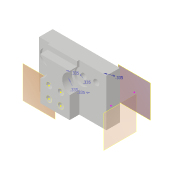
# Autodesk Inventor part: CollectorArmRollerSupportRight
Saved by Autodesk Inventor 2018 (Build 220112000, 112)
## iProperties
Created: 2018-12-16
Part Number: CollectorArmRollerSupportRight
Material: Generic
Document SubType Name: Modeling
Designer: ball
Density: 1 g/cm^3
Appearance: Default
Author: ball
Autodesk Inventor part; units mm, degrees
ref_plane "Work Plane5" through (0, 0, 0) normal (0, 0, 1) x (1, 0, 0)
sketch "Sketch1" plane through (0, 0, 0) normal (0, 0, 1) x (1, 0, 0)
  line L0 (-46.1271, -22.5825) -> (-26.1271, -22.5825) construction
  line L1 (-9.7566, 12.6962) -> (-9.7566, -12.6962) construction
  line L2 (-26.1271, 20.28) -> (-46.1271, 20.28) construction
  circle A0 centre (-49.897, 0) radius 1.778
  arc A1 (-26.7903, 1.7468) -> (-25.506, 1.3298) centre (-26.6476, 0) ccw construction
  circle A2 centre (-49.897, 0) radius 1.905
  circle A3 centre (-26.6476, 0) radius 1.905
  line L3 (-52.9366, 6.2882) -> (-52.9366, -15.9368)
  line L4 (-55.4766, 6.2882) -> (-55.4766, -15.9368) construction
  line L5 (-9.7566, -22.5825) -> (-55.4766, -22.5825)
  line L6 (-55.4766, -22.5825) -> (-55.4766, 20.28)
  line L7 (-55.4766, 20.28) -> (-9.7566, 20.28)
  line L8 (-9.7566, 20.28) -> (-9.7566, -22.5825)
  circle A4 centre (-16.5926, 2.1082) radius 2.15 construction
  circle A5 centre (-16.5926, 2.1082) radius 1.9939
  point P0 (0, 0)
  dimension "d0" = 3.81
  dimension "d1" = 3.81
  dimension "d2" = 2.54
  dimension "d3" = 3.9878
  constraints: 18 end point, 6 centre point, 3 coincident, 3 horizontal, 3 parallel, 2 point on circle, 2 vertical, 1 perpendicular, 16 other
  measures "d0" diameter of A2
  measures "d1" diameter of A3
  measures "d2" distance between parallel lines of L3 L4
  measures "d3" diameter of A5
ref_plane "Work Plane2" through (-20.9694, -2.2685, 9.225) normal (0, 0, -1) x (0.1078, 0.9942, 0)
extrude "Extrusion1" add sketch "Sketch1" along normal up to surface (9.225 mm away) contours A2 | L5 L6 L7 L8
ref_plane "Work Plane3" through (-49.3551, -24.0887, 15.745) normal (0, 0, -1) x (0, 1, 0)
ref_plane "Work Plane7" through (-55.4766, -22.5825, 9.225) normal (0, 0, 1) x (1, 0, 0)
sketch "Sketch3" plane through (-55.4766, -22.5825, 9.225) normal (0, 0, 1) x (1, 0, 0)
  line L0 (27.2386, 42.8625) -> (7.2386, 42.8625) projected
  arc A0 (27.2386, 28.0707) -> (27.2386, 14.6543) centre (29.2386, 21.3625) ccw projected
  line L1 (27.2386, 0) -> (27.2386, 14.6543) projected
  line L2 (7.2386, 14.6543) -> (7.2386, 0) projected
  line L3 (7.2386, 0) -> (27.2386, 0) projected
  arc A1 (7.2386, 14.6543) -> (7.2386, 28.0707) centre (5.2386, 21.3625) ccw projected
  line L4 (7.2386, 28.0707) -> (7.2386, 42.8625)
  line L5 (0, 42.8625) -> (45.72, 42.8625) projected
  line L6 (27.2386, 28.0707) -> (27.2386, 42.8625)
  point P0 (55.4766, 22.5825)
  constraints: 4 end point, 1 perpendicular, 1 vertical
ref_plane "Work Plane4" through (-51.466, -24.0887, 15.745) normal (0, 0, -1) x (0, 1, 0)
extrude "Extrusion3" add sketch "Sketch3" along normal up to surface (6.52 mm away)
ref_plane "Work Plane9" through (-55.4766, -22.5825, 9.225) normal (0, 0, 1) x (1, 0, 0)
sketch "Sketch4" plane through (-55.4766, -22.5825, 9.225) normal (0, 0, 1) x (1, 0, 0)
  circle A0 centre (5.5796, 22.5825) radius 1.778 projected
  circle A1 centre (5.5796, 22.5825) radius 1.905
  line L0 (7.2386, 28.0707) -> (7.2386, 42.8625) projected
  line L1 (7.2386, 42.8625) -> (0, 42.8625) projected
  line L2 (0, 42.8625) -> (0, 0) projected
  line L3 (0, 0) -> (7.2386, 0) projected
  line L4 (7.2386, 0) -> (7.2386, 14.6543) projected
  arc A2 (7.2386, 14.6543) -> (7.2386, 28.0707) centre (5.2386, 21.3625) ccw projected
  circle A3 centre (5.5796, 22.5825) radius 1.778 projected
  circle A4 centre (28.829, 22.5825) radius 1.9812 projected
  point P0 (55.4766, 22.5825)
  dimension "d18" = 3.81
  constraints: 1 centre point, 1 coincident
  measures "d18" diameter of A1
hole "Hole1" at (-49.897, 0, 9.225) at (-26.6476, 0, 9.225) direction (0, 0, -1) diameter 3.81 end through all counterbore diameter 10.16 counterbore depth 1.524
ref_plane "Work Plane8" through (-9.7566, -22.5825, 0) normal (1, 0, 0) x (0, 0, -1)
sketch "Sketch6" plane through (-9.7566, -22.5825, 0) normal (1, 0, 0) x (0, 0, -1)
  line L0 (-11.975, 30.2275) -> (-14.475, 30.2275) construction
  line L1 (-11.975, 39.7275) -> (-11.975, 30.2275) construction
  line L2 (31.025, 39.7275) -> (-11.975, 39.7275) construction
  line L3 (31.025, 38.4575) -> (-10.705, 38.4575) construction
  line L4 (-10.705, 32.1075) -> (-10.705, 28.9575) construction
  line L5 (-10.705, 28.9575) -> (-14.475, 28.9575) construction
  line L6 (-10.705, 28.9575) -> (-10.705, 32.1075)
  line L7 (0, 42.8625) -> (0, 0) projected
  line L8 (0, 32.1075) -> (0, 42.8625)
  line L9 (0, 42.8625) -> (-15.745, 42.8625)
  line L10 (-15.745, 42.8625) -> (-15.745, 28.9575)
  line L11 (-15.745, 28.9575) -> (-10.705, 28.9575)
  line L12 (3.1182, 32.1075) -> (5.3958, 32.1075) construction
  line L13 (-10.705, 32.1075) -> (0, 32.1075)
  point P0 (0, 22.5825)
  point P1 (0, 38.4575)
  dimension "d28" = 1.27
  constraints: 20 end point, 4 point on line, 3 collinear, 3 perpendicular, 1 horizontal, 2 other
  measures "d28" distance between parallel lines of L2 L3
extrude "Extrusion4" cut sketch "Sketch6" against normal through all
sketch "Sketch7" plane through (-48.238, -22.5825, 15.745) normal (0, 0, 1) x (1, 0, 0)
  circle A0 centre (6, 5.3625) radius 2 construction
  circle A1 centre (14, 5.3625) radius 2 construction
  arc A2 (7.4142, 14.7767) -> (4.5858, 11.9483) centre (6, 13.3625) ccw construction
  arc A3 (15.4142, 11.9483) -> (12.5858, 14.7767) centre (14, 13.3625) ccw construction
  point P0 (48.238, 22.5825)
sketch "Sketch9" plane through (0, 0, 0) normal (0, 0, -1) x (-1, 0, 0)
  arc A0 (43.6522, -10.6342) -> (40.8238, -7.8058) centre (42.238, -9.22) ccw construction
  arc A1 (35.6522, -7.8058) -> (32.8238, -10.6342) centre (34.238, -9.22) ccw construction
  circle A2 centre (42.238, -17.22) radius 2 construction
  circle A3 centre (34.238, -17.22) radius 2 construction
  point P0 (0, 0)
hole "Hole2" at (-34.238, -9.22, 0) at (-42.238, -9.22, 0) at (-42.238, -17.22, 0) at (-34.238, -17.22, 0) direction (0, 0, 1) diameter 3.9878 end through all
ref_plane "Work Plane6" through (0, 0, 0) normal (0, 0, -1) x (-1, 0, 0)
sketch "Sketch10" plane through (0, 0, 0) normal (0, 0, -1) x (-1, 0, 0)
  circle A0 centre (34.238, -9.22) radius 1.9939 construction
  circle A1 centre (42.238, -9.22) radius 1.9939 construction
  circle A2 centre (42.238, -17.22) radius 1.9939 construction
  circle A3 centre (34.238, -17.22) radius 1.9939 construction
  circle A4 centre (34.238, -9.22) radius 4.2545 construction
  circle A5 centre (42.238, -9.22) radius 4.2545 construction
  line L0 (34.238, -13.4745) -> (30.5535, -11.3472)
  line L1 (30.5535, -11.3472) -> (30.5535, -7.0927)
  line L2 (30.5535, -7.0927) -> (34.238, -4.9655)
  line L3 (34.238, -4.9655) -> (37.9225, -7.0927)
  line L4 (37.9225, -7.0927) -> (37.9225, -11.3472)
  line L5 (37.9225, -11.3472) -> (34.238, -13.4745)
  circle A6 centre (34.238, -17.22) radius 4.2545 construction
  circle A7 centre (42.238, -17.22) radius 4.2545 construction
  line L6 (38.4925, -17.22) -> (36.3652, -20.9045)
  line L7 (36.3652, -20.9045) -> (32.1107, -20.9045)
  line L8 (32.1107, -20.9045) -> (29.9835, -17.22)
  line L9 (29.9835, -17.22) -> (32.1107, -13.5355)
  line L10 (32.1107, -13.5355) -> (36.3652, -13.5355)
  line L11 (36.3652, -13.5355) -> (38.4925, -17.22)
  line L12 (42.238, -21.4745) -> (38.5535, -19.3472)
  line L13 (38.5535, -19.3472) -> (38.5535, -15.0927)
  line L14 (38.5535, -15.0927) -> (42.238, -12.9655)
  line L15 (42.238, -12.9655) -> (45.9225, -15.0927)
  line L16 (45.9225, -15.0927) -> (45.9225, -19.3472)
  line L17 (45.9225, -19.3472) -> (42.238, -21.4745)
  line L18 (46.4925, -9.22) -> (44.3652, -12.9045)
  line L19 (44.3652, -12.9045) -> (40.1107, -12.9045)
  line L20 (40.1107, -12.9045) -> (37.9835, -9.22)
  line L21 (37.9835, -9.22) -> (40.1107, -5.5355)
  line L22 (40.1107, -5.5355) -> (44.3652, -5.5355)
  line L23 (44.3652, -5.5355) -> (46.4925, -9.22)
  circle A8 centre (16.5926, 2.1082) radius 1.9939 construction
  circle A9 centre (16.5926, 2.1082) radius 4.2545 construction
  line L24 (16.5926, -2.1463) -> (12.9081, -0.019)
  line L25 (12.9081, -0.019) -> (12.9081, 4.2355)
  line L26 (12.9081, 4.2355) -> (16.5926, 6.3627)
  line L27 (16.5926, 6.3627) -> (20.2771, 4.2355)
  line L28 (20.2771, 4.2355) -> (20.2771, -0.019)
  line L29 (20.2771, -0.019) -> (16.5926, -2.1463)
  point P0 (0, 0)
  point P1 (42.238, -13.4745)
  dimension "d38" = 8.509
  dimension "d44" = 8.509
  dimension "d45" = 8.509
  dimension "d48" = 8.509
  dimension "d39" = 8.509
  constraints: 60 end point, 12 coincident, 3 vertical alignment, 2 point on circle, 1 centre point, 1 horizontal alignment, 73 other
  measures "d39" diameter of A5
extrude "Extrusion6" cut sketch "Sketch10" against normal blind 5.588 contours L0 L1 L2 L3 L4 L5 | L6 L7 L8 L9 L10 L11 | L12 L13 L14 L15 L16 L17 | L18 L19 L20 L21 L22 L23
extrude "Extrusion7" cut sketch "Sketch10" against normal blind 5.588 contours L24 L25 L26 L27 L28 L29
body "Solid1"
